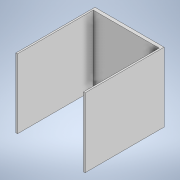
# Autodesk Inventor part: CameraHolder
Saved by Autodesk Inventor 2021.1 (Build 251245010, 245A)
## iProperties
Created: 2023-07-02
Part Number: CameraHolder
Material: Generic
Document SubType Name: Modeling
Designer: Drake
Density: 1 g/cm^3
Appearance: Default
Author: Drake
Autodesk Inventor part; units mm, degrees
ref_plane "YZ Plane" through (0, 0, 0) normal (1, 0, 0) x (0, 1, 0)
ref_plane "XZ Plane" through (0, 0, 0) normal (0, 1, 0) x (-1, 0, 0)
ref_plane "XY Plane" through (0, 0, 0) normal (0, 0, 1) x (1, 0, 0)
sketch "Sketch2" plane through (0, 0, 0) normal (0, 0, 1) x (1, 0, 0)
  line L0 (-52.5, -52.5) -> (52.5, -52.5)
  line L1 (52.5, -52.5) -> (52.5, 52.5)
  line L2 (52.5, 52.5) -> (-52.5, 52.5)
  line L3 (-52.5, 52.5) -> (-52.5, -52.5)
  line L4 (-52.5, -52.5) -> (52.5, 52.5) construction
  line L5 (52.5, -52.5) -> (-52.5, 52.5) construction
  point P0 (0, 0)
  dimension "cameraholderside" = 105
  dimension "d1" = 105
  constraints: 12 end point, 2 midpoint, 2 parallel, 1 horizontal, 1 perpendicular
  measures "cameraholderside" distance of L2.end L1.end
  measures "d1" distance of L1.end L0.end
extrude "Extrusion1" add sketch "Sketch2" along normal mid plane 120
sketch "Sketch3" plane through (0, 0, 60) normal (0, 0, 1) x (1, 0, 0)
  line L0 (-50, -57) -> (50, -57)
  line L1 (50, -57) -> (50, 57)
  line L2 (50, 57) -> (-50, 57)
  line L3 (-50, 57) -> (-50, -57)
  line L4 (-50, -57) -> (50, 57) construction
  line L5 (50, -57) -> (-50, 57) construction
  point P0 (0, 0)
  dimension "d4" = 100
  dimension "d5" = 114
  constraints: 12 end point, 2 midpoint, 2 parallel, 1 horizontal, 1 perpendicular
  measures "d4" distance of L2.end L1.end
  measures "d5" distance of L0.end L1.end
extrude "Extrusion2" cut sketch "Sketch3" against normal blind 115
body "Solid1"
